Autodesk Fusion 360 part; units mm, degrees
(part 7 of 8)
  spline S13 degree 5 poles (-13.3088, 163.635) (-13.3419, 163.5734) (-13.4079, 163.4503) (-13.5065, 163.2656) (-13.637, 163.019) (-13.7987, 162.7103) (-13.9589, 162.4013) (-14.1176, 162.0919) (-14.2748, 161.7821) (-14.4304, 161.472) (-14.5845, 161.1614) (-14.737, 160.8505) (-14.888, 160.5392) (-15.0374, 160.2275) (-15.1853, 159.9155) (-15.3315, 159.6031) (-15.4761, 159.2904) (-15.6191, 158.9773) (-15.7605, 158.6638) (-15.9002, 158.35) (-16.0383, 158.0359) (-16.1747, 157.7214) (-16.3094, 157.4066) (-16.4424, 157.0915) (-16.5736, 156.776) (-16.7032, 156.4602) (-16.831, 156.1441) (-16.957, 155.8276) (-17.0813, 155.5109) (-17.2038, 155.1938) (-17.3244, 154.8765) (-17.4432, 154.5588) (-17.5602, 154.2408) (-17.6753, 153.9225) (-17.7884, 153.604) (-17.8997, 153.2852) (-18.009, 152.966) (-18.1164, 152.6466) (-18.2218, 152.327) (-18.3252, 152.007) (-18.4266, 151.6868) (-18.5259, 151.3664) (-18.623, 151.0457) (-18.718, 150.7247) (-18.8107, 150.4035) (-18.9014, 150.0821) (-18.9898, 149.7604) (-19.0761, 149.4386) (-19.1601, 149.1164) (-19.2419, 148.7941) (-19.3211, 148.4716) (-19.3978, 148.1489) (-19.4718, 147.826) (-19.5431, 147.5028) (-19.6116, 147.1796) (-19.6777, 146.8561) (-19.7413, 146.5325) (-19.8026, 146.2087) (-19.8613, 145.8848) (-19.9172, 145.5608) (-19.9696, 145.2366) (-20.0179, 144.9123) (-20.0617, 144.588) (-20.1011, 144.2635) (-20.1367, 143.939) (-20.1694, 143.6144) (-20.1999, 143.2899) (-20.2284, 142.9653) (-20.2539, 142.6408) (-20.2738, 142.3163) (-20.2845, 141.9921) (-20.2829, 141.7329) (-20.2747, 141.5387) (-20.2659, 141.4093) (-20.2607, 141.3446) knots -1 -1 -1 -1 -1 -1 -0.98571429 -0.97142857 -0.95714286 -0.94285714 -0.92857143 -0.91428571 -0.9 -0.88571429 -0.87142857 -0.85714286 -0.84285714 -0.82857143 -0.81428571 -0.8 -0.78571429 -0.77142857 -0.75714286 -0.74285714 -0.72857143 -0.71428571 -0.7 -0.68571429 -0.67142857 -0.65714286 -0.64285714 -0.62857143 -0.61428571 -0.6 -0.58571429 -0.57142857 -0.55714286 -0.54285714 -0.52857143 -0.51428571 -0.5 -0.48571429 -0.47142857 -0.45714286 -0.44285714 -0.42857143 -0.41428571 -0.4 -0.38571429 -0.37142857 -0.35714286 -0.34285714 -0.32857143 -0.31428571 -0.3 -0.28571429 -0.27142857 -0.25714286 -0.24285714 -0.22857143 -0.21428571 -0.2 -0.18571429 -0.17142857 -0.15714286 -0.14285714 -0.12857143 -0.11428571 -0.1 -0.08571429 -0.07142857 -0.05714286 -0.04285714 -0.02857143 -0.01428571 0 0 0 0 0 0
  line L13 (-20.2607, 141.3446) -> (-19.8983, 136.8374)
  arc A27 (-21.3352, 135.1293) -> (-19.8983, 136.8374) centre (-21.4807, 136.7101) ccw
  arc A28 (-21.3352, 135.1293) -> (-31.9614, 133.7304) centre (-8.7656, -1.4025) ccw
  arc A29 (-33.7913, 135.0083) -> (-31.9614, 133.7304) centre (-32.2299, 135.295) ccw
  line L14 (-33.7913, 135.0083) -> (-34.6079, 139.4557)
  spline S14 degree 5 poles (-34.6079, 139.4557) (-34.6196, 139.5196) (-34.6446, 139.6468) (-34.687, 139.8366) (-34.7525, 140.0874) (-34.8468, 140.3978) (-34.9499, 140.706) (-35.0585, 141.0129) (-35.17, 141.319) (-35.2835, 141.6246) (-35.3991, 141.9297) (-35.5175, 142.2339) (-35.6395, 142.5371) (-35.7659, 142.8391) (-35.8964, 143.1398) (-36.0309, 143.4393) (-36.1687, 143.7379) (-36.3093, 144.0356) (-36.4523, 144.3325) (-36.5975, 144.6286) (-36.745, 144.9239) (-36.8949, 145.2184) (-37.0474, 145.5121) (-37.2024, 145.8048) (-37.36, 146.0967) (-37.5201, 146.3878) (-37.6825, 146.6779) (-37.847, 146.9673) (-38.0136, 147.2559) (-38.1823, 147.5437) (-38.3531, 147.8307) (-38.5258, 148.117) (-38.7006, 148.4024) (-38.8775, 148.6871) (-39.0563, 148.9709) (-39.2371, 149.2539) (-39.4197, 149.5362) (-39.6043, 149.8177) (-39.7907, 150.0984) (-39.9789, 150.3784) (-40.1689, 150.6576) (-40.3606, 150.936) (-40.5542, 151.2136) (-40.7494, 151.4905) (-40.9464, 151.7666) (-41.1451, 152.0419) (-41.3455, 152.3165) (-41.5475, 152.5903) (-41.7511, 152.8633) (-41.9564, 153.1356) (-42.1633, 153.4071) (-42.3717, 153.6778) (-42.5817, 153.9478) (-42.7933, 154.217) (-43.0065, 154.4855) (-43.2211, 154.7532) (-43.4373, 155.0201) (-43.655, 155.2863) (-43.8742, 155.5517) (-44.0948, 155.8164) (-44.3169, 156.0803) (-44.5404, 156.3434) (-44.7654, 156.6058) (-44.9918, 156.8674) (-45.2197, 157.1282) (-45.4489, 157.3883) (-45.6795, 157.6476) (-45.9115, 157.9062) (-46.1448, 158.164) (-46.3795, 158.421) (-46.6156, 158.6773) (-46.8055, 158.8817) (-46.9486, 159.0346) (-47.0442, 159.1365) (-47.0921, 159.1873) knots 0 0 0 0 0 0 0.01428571 0.02857143 0.04285714 0.05714286 0.07142857 0.08571429 0.1 0.11428571 0.12857143 0.14285714 0.15714286 0.17142857 0.18571429 0.2 0.21428571 0.22857143 0.24285714 0.25714286 0.27142857 0.28571429 0.3 0.31428571 0.32857143 0.34285714 0.35714286 0.37142857 0.38571429 0.4 0.41428571 0.42857143 0.44285714 0.45714286 0.47142857 0.48571429 0.5 0.51428571 0.52857143 0.54285714 0.55714286 0.57142857 0.58571429 0.6 0.61428571 0.62857143 0.64285714 0.65714286 0.67142857 0.68571429 0.7 0.71428571 0.72857143 0.74285714 0.75714286 0.77142857 0.78571429 0.8 0.81428571 0.82857143 0.84285714 0.85714286 0.87142857 0.88571429 0.9 0.91428571 0.92857143 0.94285714 0.95714286 0.97142857 0.98571429 1 1 1 1 1 1
  arc A30 (-47.0921, 159.1873) -> (-55.8688, 156.8356) centre (-8.7656, -1.4025) ccw
  spline S15 degree 5 poles (-55.8688, 156.8356) (-55.8849, 156.7676) (-55.9168, 156.6316) (-55.9642, 156.4276) (-56.0265, 156.1556) (-56.1028, 155.8157) (-56.1775, 155.4757) (-56.2507, 155.1358) (-56.3223, 154.7959) (-56.3924, 154.456) (-56.4609, 154.1162) (-56.5277, 153.7763) (-56.593, 153.4366) (-56.6567, 153.0969) (-56.7187, 152.7572) (-56.7791, 152.4176) (-56.8378, 152.0781) (-56.8949, 151.7387) (-56.9504, 151.3993) (-57.0041, 151.06) (-57.0562, 150.7209) (-57.1065, 150.3818) (-57.1551, 150.0429) (-57.202, 149.704) (-57.2472, 149.3653) (-57.2906, 149.0268) (-57.3322, 148.6883) (-57.3721, 148.3501) (-57.4101, 148.0119) (-57.4464, 147.674) (-57.4808, 147.3362) (-57.5133, 146.9986) (-57.544, 146.6612) (-57.5728, 146.324) (-57.5996, 145.987) (-57.6246, 145.6502) (-57.6476, 145.3137) (-57.6686, 144.9774) (-57.6877, 144.6413) (-57.7048, 144.3055) (-57.7198, 143.97) (-57.7328, 143.6348) (-57.7436, 143.2999) (-57.7523, 142.9653) (-57.7588, 142.631) (-57.7631, 142.2971) (-57.7653, 141.9635) (-57.7653, 141.6302) (-57.7631, 141.2973) (-57.7586, 140.9648) (-57.7517, 140.6328) (-57.7423, 140.3012) (-57.7302, 139.9701) (-57.7154, 139.6396) (-57.6979, 139.3096) (-57.678, 138.9801) (-57.6557, 138.651) (-57.6311, 138.3224) (-57.604, 137.9943) (-57.5741, 137.6669) (-57.5408, 137.3402) (-57.5035, 137.0145) (-57.4619, 136.6898) (-57.416, 136.3662) (-57.3664, 136.0436) (-57.314, 135.7216) (-57.2595, 135.4002) (-57.203, 135.0793) (-57.1436, 134.7592) (-57.0788, 134.4407) (-57.0053, 134.1247) (-56.9366, 133.8748) (-56.8784, 133.6893) (-56.8364, 133.5666) (-56.8147, 133.5054) knots -1 -1 -1 -1 -1 -1 -0.98571429 -0.97142857 -0.95714286 -0.94285714 -0.92857143 -0.91428571 -0.9 -0.88571429 -0.87142857 -0.85714286 -0.84285714 -0.82857143 -0.81428571 -0.8 -0.78571429 -0.77142857 -0.75714286 -0.74285714 -0.72857143 -0.71428571 -0.7 -0.68571429 -0.67142857 -0.65714286 -0.64285714 -0.62857143 -0.61428571 -0.6 -0.58571429 -0.57142857 -0.55714286 -0.54285714 -0.52857143 -0.51428571 -0.5 -0.48571429 -0.47142857 -0.45714286 -0.44285714 -0.42857143 -0.41428571 -0.4 -0.38571429 -0.37142857 -0.35714286 -0.34285714 -0.32857143 -0.31428571 -0.3 -0.28571429 -0.27142857 -0.25714286 -0.24285714 -0.22857143 -0.21428571 -0.2 -0.18571429 -0.17142857 -0.15714286 -0.14285714 -0.12857143 -0.11428571 -0.1 -0.08571429 -0.07142857 -0.05714286 -0.04285714 -0.02857143 -0.01428571 0 0 0 0 0 0
  line L15 (-56.8147, 133.5054) -> (-55.2981, 129.2456)
  arc A31 (-56.2439, 127.2239) -> (-55.2981, 129.2456) centre (-56.7937, 128.7131) ccw
  arc A32 (-56.2439, 127.2239) -> (-66.146, 123.1223) centre (-8.7656, -1.4025) ccw
  arc A33 (-68.2443, 123.8831) -> (-66.146, 123.1223) centre (-66.8103, 124.5641) ccw
  line L16 (-68.2443, 123.8831) -> (-70.1841, 127.9676)
  spline S16 degree 5 poles (-70.1841, 127.9676) (-70.212, 128.0263) (-70.2691, 128.1427) (-70.3591, 128.3151) (-70.4873, 128.5403) (-70.6587, 128.8157) (-70.8381, 129.0868) (-71.0224, 129.3551) (-71.2094, 129.6219) (-71.3981, 129.8878) (-71.5887, 130.1525) (-71.7818, 130.4157) (-71.9781, 130.677) (-72.1783, 130.936) (-72.3823, 131.1926) (-72.5897, 131.4472) (-72.8001, 131.6999) (-73.0129, 131.9511) (-73.2279, 132.2008) (-73.4448, 132.4493) (-73.6637, 132.6964) (-73.8848, 132.942) (-74.108, 133.1862) (-74.3336, 133.4289) (-74.5613, 133.67) (-74.7912, 133.9097) (-75.0232, 134.148) (-75.257, 134.3849) (-75.4927, 134.6206) (-75.7301, 134.8549) (-75.9693, 135.088) (-76.2103, 135.3197) (-76.453, 135.5502) (-76.6975, 135.7794) (-76.9437, 136.0072) (-77.1915, 136.2339) (-77.441, 136.4592) (-77.6922, 136.6834) (-77.9449, 136.9063) (-78.1991, 137.128) (-78.4549, 137.3485) (-78.7122, 137.5678) (-78.9709, 137.7859) (-79.2312, 138.0027) (-79.4929, 138.2185) (-79.7561, 138.433) (-80.0207, 138.6463) (-80.2867, 138.8585) (-80.5541, 139.0695) (-80.8228, 139.2794) (-81.0929, 139.4881) (-81.3644, 139.6957) (-81.6371, 139.9021) (-81.9112, 140.1074) (-82.1865, 140.3115) (-82.4632, 140.5146) (-82.7411, 140.7165) (-83.0202, 140.9172) (-83.3006, 141.1169) (-83.5822, 141.3154) (-83.865, 141.5128) (-84.1491, 141.7091) (-84.4343, 141.9043) (-84.7207, 142.0984) (-85.0083, 142.2914) (-85.297, 142.4833) (-85.5869, 142.6741) (-85.8779, 142.8638) (-86.17, 143.0524) (-86.4632, 143.2399) (-86.7576, 143.4264) (-86.9939, 143.5747) (-87.1717, 143.6854) (-87.2904, 143.759) (-87.3499, 143.7957) knots 0 0 0 0 0 0 0.01428571 0.02857143 0.04285714 0.05714286 0.07142857 0.08571429 0.1 0.11428571 0.12857143 0.14285714 0.15714286 0.17142857 0.18571429 0.2 0.21428571 0.22857143 0.24285714 0.25714286 0.27142857 0.28571429 0.3 0.31428571 0.32857143 0.34285714 0.35714286 0.37142857 0.38571429 0.4 0.41428571 0.42857143 0.44285714 0.45714286 0.47142857 0.48571429 0.5 0.51428571 0.52857143 0.54285714 0.55714286 0.57142857 0.58571429 0.6 0.61428571 0.62857143 0.64285714 0.65714286 0.67142857 0.68571429 0.7 0.71428571 0.72857143 0.74285714 0.75714286 0.77142857 0.78571429 0.8 0.81428571 0.82857143 0.84285714 0.85714286 0.87142857 0.88571429 0.9 0.91428571 0.92857143 0.94285714 0.95714286 0.97142857 0.98571429 1 1 1 1 1 1
  arc A34 (-87.3499, 143.7957) -> (-95.2189, 139.2526) centre (-8.7656, -1.4025) ccw
  spline S17 degree 5 poles (-95.2189, 139.2526) (-95.2168, 139.1827) (-95.2124, 139.0431) (-95.2054, 138.8338) (-95.1951, 138.555) (-95.1808, 138.2068) (-95.1651, 137.8591) (-95.1478, 137.5118) (-95.129, 137.165) (-95.1087, 136.8185) (-95.0869, 136.4725) (-95.0635, 136.127) (-95.0386, 135.7819) (-95.0122, 135.4373) (-94.9842, 135.0932) (-94.9546, 134.7495) (-94.9235, 134.4064) (-94.8908, 134.0637) (-94.8565, 133.7216) (-94.8206, 133.38) (-94.7831, 133.0389) (-94.744, 132.6983) (-94.7033, 132.3584) (-94.6609, 132.0189) (-94.6168, 131.6801) (-94.5711, 131.3418) (-94.5237, 131.0041) (-94.4747, 130.6671) (-94.4239, 130.3306) (-94.3714, 129.9948) (-94.3172, 129.6596) (-94.2613, 129.3251) (-94.2036, 128.9913) (-94.1441, 128.6581) (-94.0829, 128.3257) (-94.0198, 127.9939) (-93.9549, 127.6629) (-93.8882, 127.3326) (-93.8197, 127.003) (-93.7493, 126.6743) (-93.6769, 126.3463) (-93.6027, 126.0191) (-93.5264, 125.6928) (-93.4482, 125.3674) (-93.368, 125.0428) (-93.2857, 124.7191) (-93.2015, 124.3963) (-93.1153, 124.0744) (-93.027, 123.7535) (-92.9366, 123.4335) (-92.844, 123.1145) (-92.7491, 122.7967) (-92.6517, 122.48) (-92.5518, 122.1646) (-92.4496, 121.8503) (-92.3451, 121.5372) (-92.2384, 121.2251) (-92.1295, 120.9141) (-92.0185, 120.6042) (-91.9048, 120.2956) (-91.7881, 119.9887) (-91.6678, 119.6837) (-91.5436, 119.3809) (-91.4155, 119.0802) (-91.284, 118.7814) (-91.1501, 118.484) (-91.0142, 118.1876) (-90.8766, 117.8923) (-90.7364, 117.5985) (-90.5914, 117.3076) (-90.4386, 117.0214) (-90.3076, 116.7978) (-90.2033, 116.6337) (-90.131, 116.526) (-90.0942, 116.4725) knots -1 -1 -1 -1 -1 -1 -0.98571429 -0.97142857 -0.95714286 -0.94285714 -0.92857143 -0.91428571 -0.9 -0.88571429 -0.87142857 -0.85714286 -0.84285714 -0.82857143 -0.81428571 -0.8 -0.78571429 -0.77142857 -0.75714286 -0.74285714 -0.72857143 -0.71428571 -0.7 -0.68571429 -0.67142857 -0.65714286 -0.64285714 -0.62857143 -0.61428571 -0.6 -0.58571429 -0.57142857 -0.55714286 -0.54285714 -0.52857143 -0.51428571 -0.5 -0.48571429 -0.47142857 -0.45714286 -0.44285714 -0.42857143 -0.41428571 -0.4 -0.38571429 -0.37142857 -0.35714286 -0.34285714 -0.32857143 -0.31428571 -0.3 -0.28571429 -0.27142857 -0.25714286 -0.24285714 -0.22857143 -0.21428571 -0.2 -0.18571429 -0.17142857 -0.15714286 -0.14285714 -0.12857143 -0.11428571 -0.1 -0.08571429 -0.07142857 -0.05714286 -0.04285714 -0.02857143 -0.01428571 0 0 0 0 0 0
  line L17 (-90.0942, 116.4725) -> (-87.5268, 112.7504)
  arc A35 (-87.9171, 110.5527) -> (-87.5268, 112.7504) centre (-88.8336, 111.849) ccw
  arc A36 (-87.9171, 110.5527) -> (-96.4202, 104.0281) centre (-8.7656, -1.4025) ccw
  arc A37 (-98.6439, 104.2199) -> (-96.4202, 104.0281) centre (-97.4351, 105.2488) ccw
  line L18 (-98.6439, 104.2199) -> (-101.5748, 107.6632)
  spline S18 degree 5 poles (-101.5748, 107.6632) (-101.6169, 107.7126) (-101.7022, 107.8103) (-101.8337, 107.9535) (-102.0158, 108.1379) (-102.2527, 108.3596) (-102.4961, 108.5749) (-102.7436, 108.7864) (-102.9933, 108.9957) (-103.2444, 109.2037) (-103.497, 109.4101) (-103.7516, 109.6143) (-104.0089, 109.8159) (-104.2693, 110.0142) (-104.5327, 110.2094) (-104.799, 110.4016) (-105.0676, 110.5912) (-105.3382, 110.7787) (-105.6105, 110.9643) (-105.8843, 111.1482) (-106.1597, 111.3302) (-106.4368, 111.5103) (-106.7156, 111.6884) (-106.9963, 111.8644) (-107.2787, 112.0384) (-107.5628, 112.2104) (-107.8486, 112.3805) (-108.1357, 112.5488) (-108.4244, 112.7154) (-108.7144, 112.8804) (-109.0057, 113.0436) (-109.2985, 113.2051) (-109.5926, 113.3649) (-109.888, 113.5229) (-110.1848, 113.6794) (-110.4829, 113.8341) (-110.7822, 113.9872) (-111.0828, 114.1387) (-111.3846, 114.2886) (-111.6875, 114.437) (-111.9917, 114.5837) (-112.2969, 114.729) (-112.6034, 114.8726) (-112.9109, 115.0148) (-113.2195, 115.1554) (-113.5293, 115.2945) (-113.8401, 115.4321) (-114.1519, 115.5682) (-114.4648, 115.7028) (-114.7787, 115.836) (-115.0936, 115.9677) (-115.4095, 116.0979) (-115.7264, 116.2267) (-116.0443, 116.3541) (-116.3631, 116.48) (-116.6828, 116.6045) (-117.0035, 116.7276) (-117.3251, 116.8493) (-117.6476, 116.9696) (-117.971, 117.0884) (-118.2953, 117.2059) (-118.6205, 117.322) (-118.9465, 117.4368) (-119.2734, 117.5501) (-119.6011, 117.6621) (-119.9297, 117.7727) (-120.259, 117.882) (-120.5892, 117.9899) (-120.9202, 118.0965) (-121.252, 118.2018) (-121.5845, 118.3057) (-121.8512, 118.3877) (-122.0516, 118.4487) (-122.1853, 118.489) (-122.2522, 118.5091) knots 0 0 0 0 0 0 0.01428571 0.02857143 0.04285714 0.05714286 0.07142857 0.08571429 0.1 0.11428571 0.12857143 0.14285714 0.15714286 0.17142857 0.18571429 0.2 0.21428571 0.22857143 0.24285714 0.25714286 0.27142857 0.28571429 0.3 0.31428571 0.32857143 0.34285714 0.35714286 0.37142857 0.38571429 0.4 0.41428571 0.42857143 0.44285714 0.45714286 0.47142857 0.48571429 0.5 0.51428571 0.52857143 0.54285714 0.55714286 0.57142857 0.58571429 0.6 0.61428571 0.62857143 0.64285714 0.65714286 0.67142857 0.68571429 0.7 0.71428571 0.72857143 0.74285714 0.75714286 0.77142857 0.78571429 0.8 0.81428571 0.82857143 0.84285714 0.85714286 0.87142857 0.88571429 0.9 0.91428571 0.92857143 0.94285714 0.95714286 0.97142857 0.98571429 1 1 1 1 1 1
  arc A38 (-122.2522, 118.5091) -> (-128.6772, 112.0841) centre (-8.7656, -1.4025) ccw
  spline S19 degree 5 poles (-128.6772, 112.0841) (-128.6571, 112.0172) (-128.6168, 111.8835) (-128.5558, 111.6831) (-128.4738, 111.4164) (-128.3699, 111.0839) (-128.2646, 110.7521) (-128.1581, 110.4211) (-128.0501, 110.0909) (-127.9409, 109.7615) (-127.8302, 109.433) (-127.7182, 109.1053) (-127.6049, 108.7784) (-127.4902, 108.4523) (-127.3741, 108.1272) (-127.2566, 107.8029) (-127.1377, 107.4795) (-127.0174, 107.157) (-126.8957, 106.8354) (-126.7726, 106.5147) (-126.6481, 106.1949) (-126.5222, 105.8761) (-126.3949, 105.5583) (-126.2661, 105.2414) (-126.1358, 104.9255) (-126.0041, 104.6106) (-125.871, 104.2967) (-125.7363, 103.9838) (-125.6002, 103.6719) (-125.4626, 103.3611) (-125.3235, 103.0514) (-125.1829, 102.7428) (-125.0408, 102.4352) (-124.8971, 102.1288) (-124.7519, 101.8235) (-124.6051, 101.5194) (-124.4567, 101.2165) (-124.3068, 100.9147) (-124.1553, 100.6141) (-124.0022, 100.3148) (-123.8475, 100.0167) (-123.6911, 99.7199) (-123.533, 99.4244) (-123.3732, 99.1303) (-123.2117, 98.8376) (-123.0485, 98.5462) (-122.8836, 98.2562) (-122.717, 97.9676) (-122.5486, 97.6804) (-122.3785, 97.3947) (-122.2065, 97.1106) (-122.0325, 96.8282) (-121.8565, 96.5475) (-121.6784, 96.2687) (-121.4983, 95.9916) (-121.3163, 95.7162) (-121.1325, 95.4423) (-120.9468, 95.1701) (-120.7593, 94.8995) (-120.5697, 94.6309) (-120.3775, 94.3646) (-120.1824, 94.1012) (-119.984, 93.8408) (-119.7825, 93.5835) (-119.5782, 93.3289) (-119.3718, 93.0763) (-119.1639, 92.8252) (-118.9545, 92.5755) (-118.743, 92.328) (-118.5277, 92.0846) (-118.306, 91.8477) (-118.1216, 91.6656) (-117.9784, 91.5341) (-117.8807, 91.4487) (-117.8313, 91.4067) knots -1 -1 -1 -1 -1 -1 -0.98571429 -0.97142857 -0.95714286 -0.94285714 -0.92857143 -0.91428571 -0.9 -0.88571429 -0.87142857 -0.85714286 -0.84285714 -0.82857143 -0.81428571 -0.8 -0.78571429 -0.77142857 -0.75714286 -0.74285714 -0.72857143 -0.71428571 -0.7 -0.68571429 -0.67142857 -0.65714286 -0.64285714 -0.62857143 -0.61428571 -0.6 -0.58571429 -0.57142857 -0.55714286 -0.54285714 -0.52857143 -0.51428571 -0.5 -0.48571429 -0.47142857 -0.45714286 -0.44285714 -0.42857143 -0.41428571 -0.4 -0.38571429 -0.37142857 -0.35714286 -0.34285714 -0.32857143 -0.31428571 -0.3 -0.28571429 -0.27142857 -0.25714286 -0.24285714 -0.22857143 -0.21428571 -0.2 -0.18571429 -0.17142857 -0.15714286 -0.14285714 -0.12857143 -0.11428571 -0.1 -0.08571429 -0.07142857 -0.05714286 -0.04285714 -0.02857143 -0.01428571 0 0 0 0 0 0
  line L19 (-117.8313, 91.4067) -> (-114.388, 88.4758)
  arc A39 (-114.1962, 86.252) -> (-114.388, 88.4758) centre (-115.4169, 87.2669) ccw
  arc A40 (-114.1962, 86.252) -> (-120.7209, 77.749) centre (-8.7656, -1.4025) ccw
  arc A41 (-122.9185, 77.3586) -> (-120.7209, 77.749) centre (-122.0171, 78.6654) ccw
  line L20 (-122.9185, 77.3586) -> (-126.6407, 79.9261)
  spline S20 degree 5 poles (-126.6407, 79.9261) (-126.6941, 79.9629) (-126.8018, 80.0352) (-126.9659, 80.1395) (-127.1895, 80.2704) (-127.4757, 80.4233) (-127.7666, 80.5683) (-128.0604, 80.7085) (-128.3557, 80.8461) (-128.6521, 80.982) (-128.9495, 81.1159) (-129.2483, 81.2474) (-129.549, 81.3754) (-129.8518, 81.4996) (-130.1568, 81.6199) (-130.4637, 81.7367) (-130.7723, 81.8503) (-131.0822, 81.9614) (-131.3932, 82.0702) (-131.7053, 82.1769) (-132.0184, 82.2815) (-132.3327, 82.3837) (-132.6482, 82.4836) (-132.9648, 82.5809) (-133.2826, 82.6759) (-133.6016, 82.7685) (-133.9216, 82.8589) (-134.2426, 82.9472) (-134.5645, 83.0334) (-134.8873, 83.1176) (-135.2109, 83.1999) (-135.5355, 83.2801) (-135.8609, 83.3583) (-136.1872, 83.4346) (-136.5144, 83.5088) (-136.8424, 83.5811) (-137.1712, 83.6516) (-137.5007, 83.7201) (-137.831, 83.7868) (-138.162, 83.8517) (-138.4938, 83.9147) (-138.8262, 83.976) (-139.1594, 84.0355) (-139.4932, 84.0932) (-139.8278, 84.1491) (-140.1629, 84.2033) (-140.4988, 84.2558) (-140.8352, 84.3066) (-141.1723, 84.3556) (-141.5099, 84.403) (-141.8482, 84.4487) (-142.1871, 84.4927) (-142.5265, 84.5351) (-142.8665, 84.5759) (-143.207, 84.615) (-143.5481, 84.6525) (-143.8897, 84.6884) (-144.2318, 84.7227) (-144.5745, 84.7554) (-144.9176, 84.7865) (-145.2613, 84.8161) (-145.6054, 84.8441) (-145.95, 84.8705) (-146.2951, 84.8954) (-146.6407, 84.9187) (-146.9867, 84.9406) (-147.3331, 84.9609) (-147.68, 84.9797) (-148.0272, 84.9969) (-148.375, 85.0127) (-148.7231, 85.027) (-149.0019, 85.0372) (-149.2112, 85.0443) (-149.3509, 85.0486) (-149.4207, 85.0507) knots 0 0 0 0 0 0 0.01428571 0.02857143 0.04285714 0.05714286 0.07142857 0.08571429 0.1 0.11428571 0.12857143 0.14285714 0.15714286 0.17142857 0.18571429 0.2 0.21428571 0.22857143 0.24285714 0.25714286 0.27142857 0.28571429 0.3 0.31428571 0.32857143 0.34285714 0.35714286 0.37142857 0.38571429 0.4 0.41428571 0.42857143 0.44285714 0.45714286 0.47142857 0.48571429 0.5 0.51428571 0.52857143 0.54285714 0.55714286 0.57142857 0.58571429 0.6 0.61428571 0.62857143 0.64285714 0.65714286 0.67142857 0.68571429 0.7 0.71428571 0.72857143 0.74285714 0.75714286 0.77142857 0.78571429 0.8 0.81428571 0.82857143 0.84285714 0.85714286 0.87142857 0.88571429 0.9 0.91428571 0.92857143 0.94285714 0.95714286 0.97142857 0.98571429 1 1 1 1 1 1
  arc A42 (-149.4207, 85.0507) -> (-153.9639, 77.1817) centre (-8.7656, -1.4025) ccw
  spline S21 degree 5 poles (-153.9639, 77.1817) (-153.9271, 77.1223) (-153.8535, 77.0036) (-153.7428, 76.8258) (-153.5945, 76.5895) (-153.4081, 76.2951) (-153.2205, 76.0019) (-153.0319, 75.7098) (-152.8422, 75.4188) (-152.6514, 75.1289) (-152.4595, 74.8402) (-152.2665, 74.5526) (-152.0724, 74.2662) (-151.8772, 73.981) (-151.6809, 73.6969) (-151.4835, 73.4141) (-151.285, 73.1325) (-151.0853, 72.8521) (-150.8846, 72.5729) (-150.6827, 72.295) (-150.4797, 72.0184) (-150.2755, 71.743) (-150.0702, 71.469) (-149.8638, 71.1962) (-149.6562, 70.9248) (-149.4475, 70.6547) (-149.2377, 70.386) (-149.0266, 70.1186) (-148.8144, 69.8526) (-148.6011, 69.588) (-148.3866, 69.3248) (-148.1709, 69.0631) (-147.954, 68.8028) (-147.7359, 68.544) (-147.5166, 68.2868) (-147.2961, 68.031) (-147.0744, 67.7767) (-146.8515, 67.524) (-146.6274, 67.2729) (-146.402, 67.0234) (-146.1754, 66.7755) (-145.9475, 66.5293) (-145.7183, 66.2849) (-145.4878, 66.0421) (-145.2561, 65.8012) (-145.023, 65.562) (-144.7887, 65.3245) (-144.553, 65.0889) (-144.3161, 64.8551) (-144.0778, 64.6231) (-143.8382, 64.3932) (-143.597, 64.1654) (-143.3543, 63.9399) (-143.1102, 63.7166) (-142.8645, 63.4956) (-142.6174, 63.2767) (-142.3689, 63.0598) (-142.1192, 62.8448) (-141.868, 62.632) (-141.6153, 62.4216) (-141.3608, 62.2141) (-141.1041, 62.0102) (-140.8451, 61.81) (-140.5838, 61.6137) (-140.3206, 61.4206) (-140.0559, 61.23) (-139.79, 61.0413) (-139.5232, 60.8543) (-139.2549, 60.67) (-138.9839, 60.4906) (-138.7084, 60.3192) (-138.4832, 60.191) (-138.3108, 60.101) (-138.1944, 60.0438) (-138.1357, 60.016) knots -1 -1 -1 -1 -1 -1 -0.98571429 -0.97142857 -0.95714286 -0.94285714 -0.92857143 -0.91428571 -0.9 -0.88571429 -0.87142857 -0.85714286 -0.84285714 -0.82857143 -0.81428571 -0.8 -0.78571429 -0.77142857 -0.75714286 -0.74285714 -0.72857143 -0.71428571 -0.7 -0.68571429 -0.67142857 -0.65714286 -0.64285714 -0.62857143 -0.61428571 -0.6 -0.58571429 -0.57142857 -0.55714286 -0.54285714 -0.52857143 -0.51428571 -0.5 -0.48571429 -0.47142857 -0.45714286 -0.44285714 -0.42857143 -0.41428571 -0.4 -0.38571429 -0.37142857 -0.35714286 -0.34285714 -0.32857143 -0.31428571 -0.3 -0.28571429 -0.27142857 -0.25714286 -0.24285714 -0.22857143 -0.21428571 -0.2 -0.18571429 -0.17142857 -0.15714286 -0.14285714 -0.12857143 -0.11428571 -0.1 -0.08571429 -0.07142857 -0.05714286 -0.04285714 -0.02857143 -0.01428571 0 0 0 0 0 0
  line L21 (-138.1357, 60.016) -> (-134.0512, 58.0762)
  arc A43 (-133.2904, 55.9778) -> (-134.0512, 58.0762) centre (-134.7322, 56.6422) ccw
  arc A44 (-133.2904, 55.9778) -> (-137.392, 46.0758) centre (-8.7656, -1.4025) ccw
  arc A45 (-139.4137, 45.13) -> (-137.392, 46.0758) centre (-138.8813, 46.6255) ccw
  line L22 (-139.4137, 45.13) -> (-143.6736, 46.6466)
  spline S22 degree 5 poles (-143.6736, 46.6466) (-143.7347, 46.6683) (-143.8574, 46.7103) (-144.0429, 46.7685) (-144.2929, 46.8371) (-144.6088, 46.9107) (-144.9273, 46.9755) (-145.2474, 47.0349) (-145.5683, 47.0914) (-145.8897, 47.1459) (-146.2117, 47.1983) (-146.5343, 47.2479) (-146.8579, 47.2938) (-147.1826, 47.3354) (-147.5083, 47.3727) (-147.835, 47.406) (-148.1624, 47.4359) (-148.4905, 47.463) (-148.8191, 47.4876) (-149.1482, 47.5099) (-149.4777, 47.5298) (-149.8077, 47.5473) (-150.1383, 47.5621) (-150.4693, 47.5742) (-150.8009, 47.5836) (-151.133, 47.5905) (-151.4655, 47.595) (-151.7983, 47.5972) (-152.1316, 47.5972) (-152.4652, 47.595) (-152.7991, 47.5906) (-153.1334, 47.5841) (-153.468, 47.5755) (-153.8029, 47.5647) (-154.1381, 47.5517) (-154.4737, 47.5367) (-154.8094, 47.5196) (-155.1455, 47.5005) (-155.4818, 47.4795) (-155.8184, 47.4565) (-156.1551, 47.4315) (-156.4921, 47.4046) (-156.8293, 47.3759) (-157.1667, 47.3452) (-157.5043, 47.3127) (-157.8421, 47.2783) (-158.1801, 47.242) (-158.5182, 47.204) (-158.8565, 47.1641) (-159.1949, 47.1225) (-159.5335, 47.0791) (-159.8722, 47.0339) (-160.211, 46.987) (-160.5499, 46.9384) (-160.889, 46.888) (-161.2282, 46.836) (-161.5674, 46.7822) (-161.9068, 46.7268) (-162.2462, 46.6697) (-162.5857, 46.611) (-162.9253, 46.5506) (-163.265, 46.4885) (-163.6047, 46.4249) (-163.9445, 46.3596) (-164.2843, 46.2927) (-164.6241, 46.2243) (-164.964, 46.1542) (-165.3039, 46.0826) (-165.6438, 46.0094) (-165.9838, 45.9346) (-166.3238, 45.8583) (-166.5957, 45.7961) (-166.7997, 45.7487) (-166.9357, 45.7167) (-167.0037, 45.7007) knots 0 0 0 0 0 0 0.01428571 0.02857143 0.04285714 0.05714286 0.07142857 0.08571429 0.1 0.11428571 0.12857143 0.14285714 0.15714286 0.17142857 0.18571429 0.2 0.21428571 0.22857143 0.24285714 0.25714286 0.27142857 0.28571429 0.3 0.31428571 0.32857143 0.34285714 0.35714286 0.37142857 0.38571429 0.4 0.41428571 0.42857143 0.44285714 0.45714286 0.47142857 0.48571429 0.5 0.51428571 0.52857143 0.54285714 0.55714286 0.57142857 0.58571429 0.6 0.61428571 0.62857143 0.64285714 0.65714286 0.67142857 0.68571429 0.7 0.71428571 0.72857143 0.74285714 0.75714286 0.77142857 0.78571429 0.8 0.81428571 0.82857143 0.84285714 0.85714286 0.87142857 0.88571429 0.9 0.91428571 0.92857143 0.94285714 0.95714286 0.97142857 0.98571429 1 1 1 1 1 1
  arc A46 (-167.0037, 45.7007) -> (-169.3554, 36.924) centre (-8.7656, -1.4025) ccw
  spline S23 degree 5 poles (-169.3554, 36.924) (-169.3046, 36.8761) (-169.2027, 36.7805) (-169.0498, 36.6374) (-168.8454, 36.4475) (-168.5891, 36.2114) (-168.3321, 35.9767) (-168.0743, 35.7434) (-167.8157, 35.5114) (-167.5564, 35.2808) (-167.2963, 35.0515) (-167.0355, 34.8237) (-166.7739, 34.5973) (-166.5115, 34.3723) (-166.2484, 34.1488) (-165.9845, 33.9267) (-165.7198, 33.706) (-165.4544, 33.4869) (-165.1882, 33.2692) (-164.9213, 33.053) (-164.6536, 32.8384) (-164.3851, 32.6252) (-164.1159, 32.4136) (-163.8459, 32.2036) (-163.5752, 31.9951) (-163.3037, 31.7883) (-163.0314, 31.583) (-162.7584, 31.3793) (-162.4846, 31.1773) (-162.21, 30.977) (-161.9347, 30.7783) (-161.6586, 30.5813) (-161.3817, 30.386) (-161.1041, 30.1925) (-160.8257, 30.0008) (-160.5465, 29.8108) (-160.2665, 29.6226) (-159.9858, 29.4362) (-159.7043, 29.2516) (-159.4221, 29.0689) (-159.139, 28.8882) (-158.8552, 28.7093) (-158.5705, 28.5325) (-158.2851, 28.3577) (-157.9989, 28.1849) (-157.7118, 28.0142) (-157.424, 27.8455) (-157.1354, 27.6789) (-156.8461, 27.5143) (-156.5559, 27.352) (-156.2649, 27.1919) (-155.973, 27.0343) (-155.6802, 26.8793) (-155.3865, 26.7268) (-155.092, 26.5769) (-154.7967, 26.4294) (-154.5006, 26.2842) (-154.2037, 26.1412) (-153.906, 26.0006) (-153.6075, 25.8628) (-153.3079, 25.7283) (-153.0072, 25.5977) (-152.7052, 25.4714) (-152.402, 25.3494) (-152.0978, 25.231) (-151.7928, 25.1154) (-151.4871, 25.0019) (-151.181, 24.8904) (-150.8741, 24.7818) (-150.5659, 24.6786) (-150.2555, 24.5844) (-150.0047, 24.5188) (-149.815, 24.4765) (-149.6877, 24.4515) (-149.6238, 24.4398) knots -1 -1 -1 -1 -1 -1 -0.98571429 -0.97142857 -0.95714286 -0.94285714 -0.92857143 -0.91428571 -0.9 -0.88571429 -0.87142857 -0.85714286 -0.84285714 -0.82857143 -0.81428571 -0.8 -0.78571429 -0.77142857 -0.75714286 -0.74285714 -0.72857143 -0.71428571 -0.7 -0.68571429 -0.67142857 -0.65714286 -0.64285714 -0.62857143 -0.61428571 -0.6 -0.58571429 -0.57142857 -0.55714286 -0.54285714 -0.52857143 -0.51428571 -0.5 -0.48571429 -0.47142857 -0.45714286 -0.44285714 -0.42857143 -0.41428571 -0.4 -0.38571429 -0.37142857 -0.35714286 -0.34285714 -0.32857143 -0.31428571 -0.3 -0.28571429 -0.27142857 -0.25714286 -0.24285714 -0.22857143 -0.21428571 -0.2 -0.18571429 -0.17142857 -0.15714286 -0.14285714 -0.12857143 -0.11428571 -0.1 -0.08571429 -0.07142857 -0.05714286 -0.04285714 -0.02857143 -0.01428571 0 0 0 0 0 0
  line L23 (-149.6238, 24.4398) -> (-145.1764, 23.6232)
  arc A47 (-143.8985, 21.7933) -> (-145.1764, 23.6232) centre (-145.4631, 22.0618) ccw
  arc A48 (-143.8985, 21.7933) -> (-145.2974, 11.1671) centre (-8.7656, -1.4025) ccw
  arc A49 (-147.0055, 9.7302) -> (-145.2974, 11.1671) centre (-146.8783, 11.3126) ccw
  line L24 (-147.0055, 9.7302) -> (-151.5127, 10.0926)
  spline S24 degree 5 poles (-151.5127, 10.0926) (-151.5774, 10.0978) (-151.7068, 10.1065) (-151.9011, 10.1148) (-152.1602, 10.1164) (-152.4845, 10.1057) (-152.8089, 10.0858) (-153.1334, 10.0603) (-153.458, 10.0318) (-153.7826, 10.0013) (-154.1071, 9.9686) (-154.4316, 9.933) (-154.7561, 9.8936) (-155.0804, 9.8497) (-155.4047, 9.8014) (-155.7289, 9.7491) (-156.0529, 9.6932) (-156.3768, 9.6345) (-156.7006, 9.5732) (-157.0242, 9.5096) (-157.3477, 9.4435) (-157.671, 9.3749) (-157.9941, 9.3037) (-158.317, 9.2297) (-158.6397, 9.153) (-158.9622, 9.0737) (-159.2846, 8.992) (-159.6067, 8.908) (-159.9286, 8.8217) (-160.2502, 8.7333) (-160.5717, 8.6426) (-160.8929, 8.5498) (-161.2138, 8.4549) (-161.5345, 8.3577) (-161.855, 8.2585) (-162.1752, 8.1571) (-162.4951, 8.0537) (-162.8148, 7.9483) (-163.1342, 7.8409) (-163.4533, 7.7316) (-163.7721, 7.6203) (-164.0907, 7.5071) (-164.4089, 7.3921) (-164.7269, 7.2751) (-165.0446, 7.1563) (-165.3619, 7.0357) (-165.679, 6.9132) (-165.9958, 6.7889) (-166.3122, 6.6629) (-166.6283, 6.5351) (-166.9441, 6.4055) (-167.2596, 6.2742) (-167.5747, 6.1412) (-167.8896, 6.0065) (-168.204, 5.8702) (-168.5182, 5.7321) (-168.832, 5.5924) (-169.1454, 5.451) (-169.4585, 5.308) (-169.7712, 5.1634) (-170.0836, 5.0171) (-170.3957, 4.8693) (-170.7073, 4.7199) (-171.0186, 4.5689) (-171.3295, 4.4164) (-171.6401, 4.2623) (-171.9503, 4.1066) (-172.26, 3.9495) (-172.5694, 3.7908) (-172.8785, 3.6306) (-173.1871, 3.4689) (-173.4337, 3.3384) (-173.6185, 3.2398) (-173.7416, 3.1738) (-173.8031, 3.1407) knots 0 0 0 0 0 0 0.01428571 0.02857143 0.04285714 0.05714286 0.07142857 0.08571429 0.1 0.11428571 0.12857143 0.14285714 0.15714286 0.17142857 0.18571429 0.2 0.21428571 0.22857143 0.24285714 0.25714286 0.27142857 0.28571429 0.3 0.31428571 0.32857143 0.34285714 0.35714286 0.37142857 0.38571429 0.4 0.41428571 0.42857143 0.44285714 0.45714286 0.47142857 0.48571429 0.5 0.51428571 0.52857143 0.54285714 0.55714286 0.57142857 0.58571429 0.6 0.61428571 0.62857143 0.64285714 0.65714286 0.67142857 0.68571429 0.7 0.71428571 0.72857143 0.74285714 0.75714286 0.77142857 0.78571429 0.8 0.81428571 0.82857143 0.84285714 0.85714286 0.87142857 0.88571429 0.9 0.91428571 0.92857143 0.94285714 0.95714286 0.97142857 0.98571429 1 1 1 1 1 1
  arc A50 (-173.8031, 3.1407) -> (-173.8031, -5.9457) centre (-8.7656, -1.4025) ccw
  spline S25 degree 5 poles (-173.8031, -5.9457) (-173.7416, -5.9788) (-173.6185, -6.0448) (-173.4337, -6.1434) (-173.1871, -6.2739) (-172.8785, -6.4356) (-172.5694, -6.5958) (-172.26, -6.7545) (-171.9503, -6.9116) (-171.6401, -7.0673) (-171.3295, -7.2214) (-171.0186, -7.3739) (-170.7073, -7.5249) (-170.3957, -7.6743) (-170.0836, -7.8221) (-169.7712, -7.9684) (-169.4585, -8.113) (-169.1454, -8.256) (-168.832, -8.3974) (-168.5182, -8.5371) (-168.204, -8.6752) (-167.8896, -8.8115) (-167.5747, -8.9462) (-167.2596, -9.0792) (-166.9441, -9.2105) (-166.6283, -9.3401) (-166.3122, -9.4679) (-165.9958, -9.5939) (-165.679, -9.7182) (-165.3619, -9.8407) (-165.0446, -9.9613) (-164.7269, -10.0801) (-164.4089, -10.1971) (-164.0907, -10.3121) (-163.7721, -10.4253) (-163.4533, -10.5366) (-163.1342, -10.6459) (-162.8148, -10.7533) (-162.4951, -10.8587) (-162.1752, -10.9621) (-161.855, -11.0635) (-161.5345, -11.1627) (-161.2138, -11.2599) (-160.8929, -11.3548) (-160.5717, -11.4476) (-160.2502, -11.5383) (-159.9286, -11.6267) (-159.6067, -11.713) (-159.2846, -11.797) (-158.9622, -11.8787) (-158.6397, -11.958) (-158.317, -12.0347) (-157.9941, -12.1087) (-157.671, -12.1799) (-157.3477, -12.2485) (-157.0242, -12.3146) (-156.7006, -12.3782) (-156.3768, -12.4395) (-156.0529, -12.4982) (-155.7289, -12.5541) (-155.4047, -12.6064) (-155.0804, -12.6547) (-154.7561, -12.6986) (-154.4316, -12.738) (-154.1071, -12.7736) (-153.7826, -12.8063) (-153.458, -12.8368) (-153.1334, -12.8653) (-152.8089, -12.8908) (-152.4845, -12.9107) (-152.1602, -12.9214) (-151.9011, -12.9198) (-151.7068, -12.9115) (-151.5774, -12.9028) (-151.5127, -12.8976) knots -1 -1 -1 -1 -1 -1 -0.98571429 -0.97142857 -0.95714286 -0.94285714 -0.92857143 -0.91428571 -0.9 -0.88571429 -0.87142857 -0.85714286 -0.84285714 -0.82857143 -0.81428571 -0.8 -0.78571429 -0.77142857 -0.75714286 -0.74285714 -0.72857143 -0.71428571 -0.7 -0.68571429 -0.67142857 -0.65714286 -0.64285714 -0.62857143 -0.61428571 -0.6 -0.58571429 -0.57142857 -0.55714286 -0.54285714 -0.52857143 -0.51428571 -0.5 -0.48571429 -0.47142857 -0.45714286 -0.44285714 -0.42857143 -0.41428571 -0.4 -0.38571429 -0.37142857 -0.35714286 -0.34285714 -0.32857143 -0.31428571 -0.3 -0.28571429 -0.27142857 -0.25714286 -0.24285714 -0.22857143 -0.21428571 -0.2 -0.18571429 -0.17142857 -0.15714286 -0.14285714 -0.12857143 -0.11428571 -0.1 -0.08571429 -0.07142857 -0.05714286 -0.04285714 -0.02857143 -0.01428571 0 0 0 0 0 0
  line L25 (-151.5127, -12.8976) -> (-147.0055, -12.5352)
  arc A51 (-145.2974, -13.9721) -> (-147.0055, -12.5352) centre (-146.8783, -14.1176) ccw
  arc A52 (-145.2974, -13.9721) -> (-143.8985, -24.5983) centre (-8.7656, -1.4025) ccw
  arc A53 (-145.1764, -26.4282) -> (-143.8985, -24.5983) centre (-145.4631, -24.8668) ccw
  line L26 (-145.1764, -26.4282) -> (-149.6238, -27.2448)
  spline S26 degree 5 poles (-149.6238, -27.2448) (-149.6877, -27.2565) (-149.815, -27.2815) (-150.0047, -27.3238) (-150.2555, -27.3894) (-150.5659, -27.4836) (-150.8741, -27.5868) (-151.181, -27.6954) (-151.4871, -27.8069) (-151.7928, -27.9204) (-152.0978, -28.036) (-152.402, -28.1544) (-152.7052, -28.2764) (-153.0072, -28.4027) (-153.3079, -28.5333) (-153.6075, -28.6678) (-153.906, -28.8056) (-154.2037, -28.9462) (-154.5006, -29.0892) (-154.7967, -29.2344) (-155.092, -29.3819) (-155.3865, -29.5318) (-155.6802, -29.6843) (-155.973, -29.8393) (-156.2649, -29.9969) (-156.5559, -30.157) (-156.8461, -30.3193) (-157.1354, -30.4839) (-157.424, -30.6505) (-157.7118, -30.8192) (-157.9989, -30.9899) (-158.2851, -31.1627) (-158.5705, -31.3375) (-158.8552, -31.5143) (-159.139, -31.6932) (-159.4221, -31.8739) (-159.7043, -32.0566) (-159.9858, -32.2412) (-160.2665, -32.4276) (-160.5465, -32.6158) (-160.8257, -32.8058) (-161.1041, -32.9975) (-161.3817, -33.191) (-161.6586, -33.3863) (-161.9347, -33.5833) (-162.21, -33.782) (-162.4846, -33.9823) (-162.7584, -34.1843) (-163.0314, -34.388) (-163.3037, -34.5933) (-163.5752, -34.8001) (-163.8459, -35.0086) (-164.1159, -35.2186) (-164.3851, -35.4302) (-164.6536, -35.6434) (-164.9213, -35.858) (-165.1882, -36.0742) (-165.4544, -36.2919) (-165.7198, -36.511) (-165.9845, -36.7317) (-166.2484, -36.9538) (-166.5115, -37.1773) (-166.7739, -37.4023) (-167.0355, -37.6287) (-167.2963, -37.8565) (-167.5564, -38.0858) (-167.8157, -38.3164) (-168.0743, -38.5484) (-168.3321, -38.7817) (-168.5891, -39.0164) (-168.8454, -39.2525) (-169.0498, -39.4424) (-169.2027, -39.5855) (-169.3046, -39.6811) (-169.3554, -39.729) knots 0 0 0 0 0 0 0.01428571 0.02857143 0.04285714 0.05714286 0.07142857 0.08571429 0.1 0.11428571 0.12857143 0.14285714 0.15714286 0.17142857 0.18571429 0.2 0.21428571 0.22857143 0.24285714 0.25714286 0.27142857 0.28571429 0.3 0.31428571 0.32857143 0.34285714 0.35714286 0.37142857 0.38571429 0.4 0.41428571 0.42857143 0.44285714 0.45714286 0.47142857 0.48571429 0.5 0.51428571 0.52857143 0.54285714 0.55714286 0.57142857 0.58571429 0.6 0.61428571 0.62857143 0.64285714 0.65714286 0.67142857 0.68571429 0.7 0.71428571 0.72857143 0.74285714 0.75714286 0.77142857 0.78571429 0.8 0.81428571 0.82857143 0.84285714 0.85714286 0.87142857 0.88571429 0.9 0.91428571 0.92857143 0.94285714 0.95714286 0.97142857 0.98571429 1 1 1 1 1 1
  arc A54 (-169.3554, -39.729) -> (-167.0037, -48.5057) centre (-8.7656, -1.4025) ccw
  spline S27 degree 5 poles (-167.0037, -48.5057) (-166.9357, -48.5217) (-166.7997, -48.5537) (-166.5957, -48.6011) (-166.3238, -48.6633) (-165.9838, -48.7396) (-165.6438, -48.8144) (-165.3039, -48.8876) (-164.964, -48.9592) (-164.6241, -49.0293) (-164.2843, -49.0977) (-163.9445, -49.1646) (-163.6047, -49.2299) (-163.265, -49.2935) (-162.9253, -49.3556) (-162.5857, -49.416) (-162.2462, -49.4747) (-161.9068, -49.5318) (-161.5674, -49.5872) (-161.2282, -49.641) (-160.889, -49.693) (-160.5499, -49.7434) (-160.211, -49.792) (-159.8722, -49.8389) (-159.5335, -49.8841) (-159.1949, -49.9275) (-158.8565, -49.9691) (-158.5182, -50.009) (-158.1801, -50.047) (-157.8421, -50.0832) (-157.5043, -50.1176) (-157.1667, -50.1502) (-156.8293, -50.1809) (-156.4921, -50.2096) (-156.1551, -50.2365) (-155.8184, -50.2615) (-155.4818, -50.2845) (-155.1455, -50.3055) (-154.8094, -50.3246) (-154.4737, -50.3417) (-154.1381, -50.3567) (-153.8029, -50.3697) (-153.468, -50.3805) (-153.1334, -50.3891) (-152.7991, -50.3956) (-152.4652, -50.4) (-152.1316, -50.4022) (-151.7983, -50.4022) (-151.4655, -50.4) (-151.133, -50.3955) (-150.8009, -50.3886) (-150.4693, -50.3792) (-150.1383, -50.3671) (-149.8077, -50.3523) (-149.4777, -50.3348) (-149.1482, -50.3149) (-148.8191, -50.2926) (-148.4905, -50.268) (-148.1624, -50.2409) (-147.835, -50.211) (-147.5083, -50.1777) (-147.1826, -50.1404) (-146.8579, -50.0988) (-146.5343, -50.0529) (-146.2117, -50.0033) (-145.8897, -49.9509) (-145.5683, -49.8963) (-145.2474, -49.8399) (-144.9273, -49.7805) (-144.6088, -49.7157) (-144.2929, -49.6421) (-144.0429, -49.5735) (-143.8574, -49.5153) (-143.7347, -49.4733) (-143.6736, -49.4516) knots -1 -1 -1 -1 -1 -1 -0.98571429 -0.97142857 -0.95714286 -0.94285714 -0.92857143 -0.91428571 -0.9 -0.88571429 -0.87142857 -0.85714286 -0.84285714 -0.82857143 -0.81428571 -0.8 -0.78571429 -0.77142857 -0.75714286 -0.74285714 -0.72857143 -0.71428571 -0.7 -0.68571429 -0.67142857 -0.65714286 -0.64285714 -0.62857143 -0.61428571 -0.6 -0.58571429 -0.57142857 -0.55714286 -0.54285714 -0.52857143 -0.51428571 -0.5 -0.48571429 -0.47142857 -0.45714286 -0.44285714 -0.42857143 -0.41428571 -0.4 -0.38571429 -0.37142857 -0.35714286 -0.34285714 -0.32857143 -0.31428571 -0.3 -0.28571429 -0.27142857 -0.25714286 -0.24285714 -0.22857143 -0.21428571 -0.2 -0.18571429 -0.17142857 -0.15714286 -0.14285714 -0.12857143 -0.11428571 -0.1 -0.08571429 -0.07142857 -0.05714286 -0.04285714 -0.02857143 -0.01428571 0 0 0 0 0 0
  line L27 (-143.6736, -49.4516) -> (-139.4137, -47.935)
  arc A55 (-137.392, -48.8808) -> (-139.4137, -47.935) centre (-138.8813, -49.4305) ccw
  arc A56 (-137.392, -48.8808) -> (-133.2904, -58.7828) centre (-8.7656, -1.4025) ccw
  arc A57 (-134.0512, -60.8812) -> (-133.2904, -58.7828) centre (-134.7322, -59.4472) ccw
  line L28 (-134.0512, -60.8812) -> (-138.1357, -62.821)
  spline S28 degree 5 poles (-138.1357, -62.821) (-138.1944, -62.8488) (-138.3108, -62.906) (-138.4832, -62.996) (-138.7084, -63.1242) (-138.9839, -63.2956) (-139.2549, -63.475) (-139.5232, -63.6593) (-139.79, -63.8463) (-140.0559, -64.035) (-140.3206, -64.2256) (-140.5838, -64.4187) (-140.8451, -64.615) (-141.1041, -64.8152) (-141.3608, -65.0191) (-141.6153, -65.2266) (-141.868, -65.437) (-142.1192, -65.6498) (-142.3689, -65.8648) (-142.6174, -66.0817) (-142.8645, -66.3006) (-143.1102, -66.5216) (-143.3543, -66.7449) (-143.597, -66.9704) (-143.8382, -67.1982) (-144.0778, -67.4281) (-144.3161, -67.6601) (-144.553, -67.8939) (-144.7887, -68.1295) (-145.023, -68.367) (-145.2561, -68.6062) (-145.4878, -68.8471) (-145.7183, -69.0899) (-145.9475, -69.3343) (-146.1754, -69.5805) (-146.402, -69.8284) (-146.6274, -70.0779) (-146.8515, -70.329) (-147.0744, -70.5817) (-147.2961, -70.836) (-147.5166, -71.0918) (-147.7359, -71.349) (-147.954, -71.6078) (-148.1709, -71.8681) (-148.3866, -72.1298) (-148.6011, -72.393) (-148.8144, -72.6576) (-149.0266, -72.9236) (-149.2377, -73.191) (-149.4475, -73.4597) (-149.6562, -73.7298) (-149.8638, -74.0012) (-150.0702, -74.274) (-150.2755, -74.548) (-150.4797, -74.8234) (-150.6827, -75.1) (-150.8846, -75.3779) (-151.0853, -75.6571) (-151.285, -75.9375) (-151.4835, -76.2191) (-151.6809, -76.5019) (-151.8772, -76.786) (-152.0724, -77.0712) (-152.2665, -77.3576) (-152.4595, -77.6452) (-152.6514, -77.9339) (-152.8422, -78.2238) (-153.0319, -78.5148) (-153.2205, -78.8069) (-153.4081, -79.1001) (-153.5945, -79.3945) (-153.7428, -79.6308) (-153.8535, -79.8086) (-153.9271, -79.9273) (-153.9639, -79.9867) knots 0 0 0 0 0 0 0.01428571 0.02857143 0.04285714 0.05714286 0.07142857 0.08571429 0.1 0.11428571 0.12857143 0.14285714 0.15714286 0.17142857 0.18571429 0.2 0.21428571 0.22857143 0.24285714 0.25714286 0.27142857 0.28571429 0.3 0.31428571 0.32857143 0.34285714 0.35714286 0.37142857 0.38571429 0.4 0.41428571 0.42857143 0.44285714 0.45714286 0.47142857 0.48571429 0.5 0.51428571 0.52857143 0.54285714 0.55714286 0.57142857 0.58571429 0.6 0.61428571 0.62857143 0.64285714 0.65714286 0.67142857 0.68571429 0.7 0.71428571 0.72857143 0.74285714 0.75714286 0.77142857 0.78571429 0.8 0.81428571 0.82857143 0.84285714 0.85714286 0.87142857 0.88571429 0.9 0.91428571 0.92857143 0.94285714 0.95714286 0.97142857 0.98571429 1 1 1 1 1 1
  arc A58 (-153.9639, -79.9867) -> (-149.4207, -87.8557) centre (-8.7656, -1.4025) ccw
  spline S29 degree 5 poles (-149.4207, -87.8557) (-149.3509, -87.8536) (-149.2112, -87.8493) (-149.0019, -87.8422) (-148.7231, -87.832) (-148.375, -87.8177) (-148.0272, -87.8019) (-147.68, -87.7847) (-147.3331, -87.7659) (-146.9867, -87.7456) (-146.6407, -87.7237) (-146.2951, -87.7004) (-145.95, -87.6755) (-145.6054, -87.6491) (-145.2613, -87.6211) (-144.9176, -87.5915) (-144.5745, -87.5604) (-144.2318, -87.5277) (-143.8897, -87.4934) (-143.5481, -87.4575) (-143.207, -87.42) (-142.8665, -87.3809) (-142.5265, -87.3401) (-142.1871, -87.2977) (-141.8482, -87.2537) (-141.5099, -87.208) (-141.1723, -87.1606) (-140.8352, -87.1116) (-140.4988, -87.0608) (-140.1629, -87.0083) (-139.8278, -86.9541) (-139.4932, -86.8982) (-139.1594, -86.8405) (-138.8262, -86.781) (-138.4938, -86.7197) (-138.162, -86.6567) (-137.831, -86.5918) (-137.5007, -86.5251) (-137.1712, -86.4566) (-136.8424, -86.3861) (-136.5144, -86.3138) (-136.1872, -86.2396) (-135.8609, -86.1633) (-135.5355, -86.0851) (-135.2109, -86.0049) (-134.8873, -85.9226) (-134.5645, -85.8384) (-134.2426, -85.7522) (-133.9216, -85.6639) (-133.6016, -85.5735) (-133.2826, -85.4809) (-132.9648, -85.3859) (-132.6482, -85.2886) (-132.3327, -85.1887) (-132.0184, -85.0865) (-131.7053, -84.9819) (-131.3932, -84.8752) (-131.0822, -84.7664) (-130.7723, -84.6553) (-130.4637, -84.5417) (-130.1568, -84.4249) (-129.8518, -84.3046) (-129.549, -84.1804) (-129.2483, -84.0524) (-128.9495, -83.9209) (-128.6521, -83.7869) (-128.3557, -83.6511) (-128.0604, -83.5135) (-127.7666, -83.3733) (-127.4757, -83.2283) (-127.1895, -83.0754) (-126.9659, -82.9445) (-126.8018, -82.8402) (-126.6941, -82.7679) (-126.6407, -82.7311) knots -1 -1 -1 -1 -1 -1 -0.98571429 -0.97142857 -0.95714286 -0.94285714 -0.92857143 -0.91428571 -0.9 -0.88571429 -0.87142857 -0.85714286 -0.84285714 -0.82857143 -0.81428571 -0.8 -0.78571429 -0.77142857 -0.75714286 -0.74285714 -0.72857143 -0.71428571 -0.7 -0.68571429 -0.67142857 -0.65714286 -0.64285714 -0.62857143 -0.61428571 -0.6 -0.58571429 -0.57142857 -0.55714286 -0.54285714 -0.52857143 -0.51428571 -0.5 -0.48571429 -0.47142857 -0.45714286 -0.44285714 -0.42857143 -0.41428571 -0.4 -0.38571429 -0.37142857 -0.35714286 -0.34285714 -0.32857143 -0.31428571 -0.3 -0.28571429 -0.27142857 -0.25714286 -0.24285714 -0.22857143 -0.21428571 -0.2 -0.18571429 -0.17142857 -0.15714286 -0.14285714 -0.12857143 -0.11428571 -0.1 -0.08571429 -0.07142857 -0.05714286 -0.04285714 -0.02857143 -0.01428571 0 0 0 0 0 0
  line L29 (-126.6407, -82.7311) -> (-122.9185, -80.1636)
  arc A59 (-120.7209, -80.554) -> (-122.9185, -80.1636) centre (-122.0171, -81.4704) ccw
  arc A60 (-120.7209, -80.554) -> (-114.1962, -89.057) centre (-8.7656, -1.4025) ccw
  arc A61 (-114.388, -91.2808) -> (-114.1962, -89.057) centre (-115.4169, -90.0719) ccw
  line L30 (-114.388, -91.2808) -> (-117.8313, -94.2117)
  spline S30 degree 5 poles (-117.8313, -94.2117) (-117.8807, -94.2537) (-117.9784, -94.3391) (-118.1216, -94.4706) (-118.306, -94.6527) (-118.5277, -94.8896) (-118.743, -95.133) (-118.9545, -95.3805) (-119.1639, -95.6302) (-119.3718, -95.8813) (-119.5782, -96.1339) (-119.7825, -96.3885) (-119.984, -96.6458) (-120.1824, -96.9062) (-120.3775, -97.1696) (-120.5697, -97.4359) (-120.7593, -97.7045) (-120.9468, -97.9751) (-121.1325, -98.2473) (-121.3163, -98.5212) (-121.4983, -98.7966) (-121.6784, -99.0737) (-121.8565, -99.3525) (-122.0325, -99.6332) (-122.2065, -99.9156) (-122.3785, -100.1997) (-122.5486, -100.4854) (-122.717, -100.7726) (-122.8836, -101.0612) (-123.0485, -101.3512) (-123.2117, -101.6426) (-123.3732, -101.9353) (-123.533, -102.2294) (-123.6911, -102.5249) (-123.8475, -102.8217) (-124.0022, -103.1198) (-124.1553, -103.4191) (-124.3068, -103.7197) (-124.4567, -104.0215) (-124.6051, -104.3244) (-124.7519, -104.6285) (-124.8971, -104.9338) (-125.0408, -105.2402) (-125.1829, -105.5478) (-125.3235, -105.8564) (-125.4626, -106.1661) (-125.6002, -106.4769) (-125.7363, -106.7888) (-125.871, -107.1017) (-126.0041, -107.4156) (-126.1358, -107.7305) (-126.2661, -108.0464) (-126.3949, -108.3633) (-126.5222, -108.6811) (-126.6481, -108.9999) (-126.7726, -109.3197) (-126.8957, -109.6404) (-127.0174, -109.962) (-127.1377, -110.2845) (-127.2566, -110.6079) (-127.3741, -110.9322) (-127.4902, -111.2573) (-127.6049, -111.5834) (-127.7182, -111.9103) (-127.8302, -112.238) (-127.9409, -112.5665) (-128.0501, -112.8959) (-128.1581, -113.2261) (-128.2646, -113.5571) (-128.3699, -113.8889) (-128.4738, -114.2214) (-128.5558, -114.4881) (-128.6168, -114.6885) (-128.6571, -114.8222) (-128.6772, -114.8891) knots 0 0 0 0 0 0 0.01428571 0.02857143 0.04285714 0.05714286 0.07142857 0.08571429 0.1 0.11428571 0.12857143 0.14285714 0.15714286 0.17142857 0.18571429 0.2 0.21428571 0.22857143 0.24285714 0.25714286 0.27142857 0.28571429 0.3 0.31428571 0.32857143 0.34285714 0.35714286 0.37142857 0.38571429 0.4 0.41428571 0.42857143 0.44285714 0.45714286 0.47142857 0.48571429 0.5 0.51428571 0.52857143 0.54285714 0.55714286 0.57142857 0.58571429 0.6 0.61428571 0.62857143 0.64285714 0.65714286 0.67142857 0.68571429 0.7 0.71428571 0.72857143 0.74285714 0.75714286 0.77142857 0.78571429 0.8 0.81428571 0.82857143 0.84285714 0.85714286 0.87142857 0.88571429 0.9 0.91428571 0.92857143 0.94285714 0.95714286 0.97142857 0.98571429 1 1 1 1 1 1
  arc A62 (-128.6772, -114.8891) -> (-122.2522, -121.3141) centre (-8.7656, -1.4025) ccw
  spline S31 degree 5 poles (-122.2522, -121.3141) (-122.1853, -121.294) (-122.0516, -121.2537) (-121.8512, -121.1927) (-121.5845, -121.1107) (-121.252, -121.0068) (-120.9202, -120.9015) (-120.5892, -120.7949) (-120.259, -120.687) (-119.9297, -120.5777) (-119.6011, -120.4671) (-119.2734, -120.3551) (-118.9465, -120.2418) (-118.6205, -120.127) (-118.2953, -120.0109) (-117.971, -119.8934) (-117.6476, -119.7746) (-117.3251, -119.6543) (-117.0035, -119.5326) (-116.6828, -119.4095) (-116.3631, -119.285) (-116.0443, -119.1591) (-115.7264, -119.0317) (-115.4095, -118.9029) (-115.0936, -118.7727) (-114.7787, -118.641) (-114.4648, -118.5078) (-114.1519, -118.3732) (-113.8401, -118.2371) (-113.5293, -118.0995) (-113.2195, -117.9604) (-112.9109, -117.8198) (-112.6034, -117.6776) (-112.2969, -117.534) (-111.9917, -117.3887) (-111.6875, -117.242) (-111.3846, -117.0936) (-111.0828, -116.9437) (-110.7822, -116.7922) (-110.4829, -116.6391) (-110.1848, -116.4843) (-109.888, -116.3279) (-109.5926, -116.1699) (-109.2985, -116.0101) (-109.0057, -115.8486) (-108.7144, -115.6854) (-108.4244, -115.5204) (-108.1357, -115.3538) (-107.8486, -115.1855) (-107.5628, -115.0154) (-107.2787, -114.8434) (-106.9963, -114.6694) (-106.7156, -114.4934) (-106.4368, -114.3153) (-106.1597, -114.1352) (-105.8843, -113.9532) (-105.6105, -113.7693) (-105.3382, -113.5837) (-105.0676, -113.3962) (-104.799, -113.2066) (-104.5327, -113.0144) (-104.2693, -112.8192) (-104.0089, -112.6209) (-103.7516, -112.4193) (-103.497, -112.215) (-103.2444, -112.0087) (-102.9933, -111.8007) (-102.7436, -111.5914) (-102.4961, -111.3799) (-102.2527, -111.1646) (-102.0158, -110.9429) (-101.8337, -110.7585) (-101.7022, -110.6153) (-101.6169, -110.5176) (-101.5748, -110.4682) knots -1 -1 -1 -1 -1 -1 -0.98571429 -0.97142857 -0.95714286 -0.94285714 -0.92857143 -0.91428571 -0.9 -0.88571429 -0.87142857 -0.85714286 -0.84285714 -0.82857143 -0.81428571 -0.8 -0.78571429 -0.77142857 -0.75714286 -0.74285714 -0.72857143 -0.71428571 -0.7 -0.68571429 -0.67142857 -0.65714286 -0.64285714 -0.62857143 -0.61428571 -0.6 -0.58571429 -0.57142857 -0.55714286 -0.54285714 -0.52857143 -0.51428571 -0.5 -0.48571429 -0.47142857 -0.45714286 -0.44285714 -0.42857143 -0.41428571 -0.4 -0.38571429 -0.37142857 -0.35714286 -0.34285714 -0.32857143 -0.31428571 -0.3 -0.28571429 -0.27142857 -0.25714286 -0.24285714 -0.22857143 -0.21428571 -0.2 -0.18571429 -0.17142857 -0.15714286 -0.14285714 -0.12857143 -0.11428571 -0.1 -0.08571429 -0.07142857 -0.05714286 -0.04285714 -0.02857143 -0.01428571 0 0 0 0 0 0
  line L31 (-101.5748, -110.4682) -> (-98.6439, -107.0249)
  arc A63 (-96.4202, -106.8331) -> (-98.6439, -107.0249) centre (-97.4351, -108.0538) ccw
  arc A64 (-96.4202, -106.8331) -> (-87.9171, -113.3577) centre (-8.7656, -1.4025) ccw
  arc A65 (-87.5268, -115.5554) -> (-87.9171, -113.3577) centre (-88.8336, -114.654) ccw
  line L32 (-87.5268, -115.5554) -> (-90.0942, -119.2775)